Autodesk Fusion 360 part; units mm, degrees
(part 5 of 6)
  spline S27 degree 5 poles (67.7388, 69.1152) (67.7383, 69.1039) (67.7372, 69.0814) (67.7356, 69.0477) (67.7337, 69.0027) (67.7316, 68.9466) (67.7297, 68.8905) (67.728, 68.8344) (67.7266, 68.7785) (67.7254, 68.7226) (67.7245, 68.6668) (67.7239, 68.611) (67.7235, 68.5553) (67.7233, 68.4997) (67.7234, 68.4441) (67.7237, 68.3886) (67.7243, 68.3332) (67.7252, 68.2779) (67.7263, 68.2226) (67.7277, 68.1674) (67.7294, 68.1123) (67.7313, 68.0573) (67.7334, 68.0023) (67.7359, 67.9474) (67.7386, 67.8927) (67.7416, 67.838) (67.7448, 67.7833) (67.7484, 67.7288) (67.7522, 67.6744) (67.7562, 67.6201) (67.7606, 67.5658) (67.7652, 67.5117) (67.7702, 67.4576) (67.7754, 67.4037) (67.7809, 67.3498) (67.7867, 67.2961) (67.7928, 67.2424) (67.7992, 67.1889) (67.8059, 67.1355) (67.8129, 67.0822) (67.8202, 67.029) (67.8278, 66.9759) (67.8357, 66.923) (67.844, 66.8701) (67.8526, 66.8174) (67.8615, 66.7649) (67.8707, 66.7124) (67.8803, 66.6601) (67.8901, 66.6079) (67.9004, 66.5559) (67.9109, 66.504) (67.9219, 66.4523) (67.9333, 66.4007) (67.945, 66.3493) (67.9572, 66.2981) (67.9697, 66.247) (67.9825, 66.1961) (67.9957, 66.1454) (68.0093, 66.0948) (68.0233, 66.0444) (68.0378, 65.9942) (68.0528, 65.9443) (68.0685, 65.8947) (68.0848, 65.8454) (68.1017, 65.7964) (68.1189, 65.7475) (68.1365, 65.6989) (68.1543, 65.6503) (68.1726, 65.602) (68.1917, 65.5541) (68.212, 65.5069) (68.2297, 65.4698) (68.2439, 65.4424) (68.2539, 65.4245) (68.2589, 65.4155) knots -1 -1 -1 -1 -1 -1 -0.98571429 -0.97142857 -0.95714286 -0.94285714 -0.92857143 -0.91428571 -0.9 -0.88571429 -0.87142857 -0.85714286 -0.84285714 -0.82857143 -0.81428571 -0.8 -0.78571429 -0.77142857 -0.75714286 -0.74285714 -0.72857143 -0.71428571 -0.7 -0.68571429 -0.67142857 -0.65714286 -0.64285714 -0.62857143 -0.61428571 -0.6 -0.58571429 -0.57142857 -0.55714286 -0.54285714 -0.52857143 -0.51428571 -0.5 -0.48571429 -0.47142857 -0.45714286 -0.44285714 -0.42857143 -0.41428571 -0.4 -0.38571429 -0.37142857 -0.35714286 -0.34285714 -0.32857143 -0.31428571 -0.3 -0.28571429 -0.27142857 -0.25714286 -0.24285714 -0.22857143 -0.21428571 -0.2 -0.18571429 -0.17142857 -0.15714286 -0.14285714 -0.12857143 -0.11428571 -0.1 -0.08571429 -0.07142857 -0.05714286 -0.04285714 -0.02857143 -0.01428571 0 0 0 0 0 0
  line L29 (68.2589, 65.4155) -> (68.5051, 64.9824)
  arc A61 (68.3271, 64.3063) -> (68.5051, 64.9824) centre (68.0704, 64.7354) ccw
  arc A62 (68.3271, 64.3063) -> (67.3329, 63.6754) centre (79.882, 45) ccw
  arc A63 (66.6454, 63.8023) -> (67.3329, 63.6754) centre (67.0541, 64.0904) ccw
  line L30 (66.6454, 63.8023) -> (66.3584, 64.2094)
  spline S28 degree 5 poles (66.3584, 64.2094) (66.3524, 64.2178) (66.3404, 64.2344) (66.3217, 64.2589) (66.2957, 64.2907) (66.2616, 64.3293) (66.2264, 64.3669) (66.1905, 64.404) (66.1541, 64.4408) (66.1175, 64.4774) (66.0807, 64.5138) (66.0435, 64.55) (66.0058, 64.5857) (65.9676, 64.621) (65.9289, 64.6559) (65.8897, 64.6904) (65.85, 64.7245) (65.81, 64.7583) (65.7697, 64.7919) (65.7291, 64.8252) (65.6883, 64.8582) (65.6471, 64.891) (65.6056, 64.9235) (65.5638, 64.9558) (65.5216, 64.9877) (65.4792, 65.0194) (65.4365, 65.0508) (65.3935, 65.0819) (65.3502, 65.1129) (65.3067, 65.1435) (65.2629, 65.174) (65.2189, 65.2042) (65.1746, 65.2341) (65.1301, 65.2639) (65.0853, 65.2934) (65.0403, 65.3226) (64.995, 65.3516) (64.9495, 65.3804) (64.9038, 65.409) (64.8579, 65.4374) (64.8117, 65.4655) (64.7653, 65.4934) (64.7187, 65.5211) (64.6719, 65.5486) (64.6249, 65.5758) (64.5777, 65.6029) (64.5303, 65.6297) (64.4826, 65.6563) (64.4348, 65.6827) (64.3868, 65.7089) (64.3385, 65.7349) (64.2901, 65.7607) (64.2415, 65.7863) (64.1927, 65.8116) (64.1437, 65.8368) (64.0946, 65.8617) (64.0452, 65.8865) (63.9957, 65.911) (63.946, 65.9354) (63.8961, 65.9595) (63.8461, 65.9835) (63.7958, 66.0072) (63.7454, 66.0308) (63.6948, 66.0541) (63.6441, 66.0772) (63.5932, 66.1002) (63.5421, 66.1229) (63.4909, 66.1455) (63.4395, 66.1678) (63.3879, 66.19) (63.3362, 66.212) (63.2947, 66.2294) (63.2635, 66.2423) (63.2427, 66.2509) (63.2322, 66.2552) knots 0 0 0 0 0 0 0.01428571 0.02857143 0.04285714 0.05714286 0.07142857 0.08571429 0.1 0.11428571 0.12857143 0.14285714 0.15714286 0.17142857 0.18571429 0.2 0.21428571 0.22857143 0.24285714 0.25714286 0.27142857 0.28571429 0.3 0.31428571 0.32857143 0.34285714 0.35714286 0.37142857 0.38571429 0.4 0.41428571 0.42857143 0.44285714 0.45714286 0.47142857 0.48571429 0.5 0.51428571 0.52857143 0.54285714 0.55714286 0.57142857 0.58571429 0.6 0.61428571 0.62857143 0.64285714 0.65714286 0.67142857 0.68571429 0.7 0.71428571 0.72857143 0.74285714 0.75714286 0.77142857 0.78571429 0.8 0.81428571 0.82857143 0.84285714 0.85714286 0.87142857 0.88571429 0.9 0.91428571 0.92857143 0.94285714 0.95714286 0.97142857 0.98571429 1 1 1 1 1 1
  arc A64 (63.2322, 66.2552) -> (62.1231, 65.3377) centre (79.882, 45) ccw
  spline S29 degree 5 poles (62.1231, 65.3377) (62.1254, 65.3266) (62.1299, 65.3046) (62.1368, 65.2715) (62.1462, 65.2275) (62.158, 65.1725) (62.1701, 65.1177) (62.1825, 65.0631) (62.195, 65.0085) (62.2078, 64.9541) (62.2208, 64.8998) (62.234, 64.8456) (62.2475, 64.7915) (62.2612, 64.7376) (62.2751, 64.6838) (62.2892, 64.6302) (62.3036, 64.5766) (62.3182, 64.5233) (62.333, 64.47) (62.3481, 64.4169) (62.3634, 64.3639) (62.3789, 64.3111) (62.3947, 64.2584) (62.4107, 64.2059) (62.4269, 64.1535) (62.4434, 64.1013) (62.4601, 64.0492) (62.4771, 63.9972) (62.4943, 63.9455) (62.5118, 63.8938) (62.5295, 63.8424) (62.5475, 63.7911) (62.5657, 63.74) (62.5842, 63.689) (62.6029, 63.6382) (62.6219, 63.5876) (62.6411, 63.5372) (62.6606, 63.4869) (62.6804, 63.4368) (62.7004, 63.387) (62.7207, 63.3372) (62.7413, 63.2877) (62.7622, 63.2384) (62.7833, 63.1893) (62.8047, 63.1404) (62.8264, 63.0917) (62.8484, 63.0432) (62.8707, 62.9949) (62.8932, 62.9468) (62.9161, 62.899) (62.9392, 62.8513) (62.9627, 62.804) (62.9865, 62.7568) (63.0107, 62.71) (63.0352, 62.6634) (63.06, 62.6171) (63.0851, 62.5709) (63.1105, 62.5251) (63.1362, 62.4794) (63.1623, 62.4341) (63.1888, 62.3891) (63.2158, 62.3445) (63.2434, 62.3004) (63.2714, 62.2567) (63.2999, 62.2134) (63.3288, 62.1704) (63.3579, 62.1276) (63.3873, 62.085) (63.417, 62.0427) (63.4473, 62.0011) (63.4788, 61.9604) (63.5052, 61.9289) (63.5257, 61.9059) (63.5398, 61.891) (63.547, 61.8836) knots -1 -1 -1 -1 -1 -1 -0.98571429 -0.97142857 -0.95714286 -0.94285714 -0.92857143 -0.91428571 -0.9 -0.88571429 -0.87142857 -0.85714286 -0.84285714 -0.82857143 -0.81428571 -0.8 -0.78571429 -0.77142857 -0.75714286 -0.74285714 -0.72857143 -0.71428571 -0.7 -0.68571429 -0.67142857 -0.65714286 -0.64285714 -0.62857143 -0.61428571 -0.6 -0.58571429 -0.57142857 -0.55714286 -0.54285714 -0.52857143 -0.51428571 -0.5 -0.48571429 -0.47142857 -0.45714286 -0.44285714 -0.42857143 -0.41428571 -0.4 -0.38571429 -0.37142857 -0.35714286 -0.34285714 -0.32857143 -0.31428571 -0.3 -0.28571429 -0.27142857 -0.25714286 -0.24285714 -0.22857143 -0.21428571 -0.2 -0.18571429 -0.17142857 -0.15714286 -0.14285714 -0.12857143 -0.11428571 -0.1 -0.08571429 -0.07142857 -0.05714286 -0.04285714 -0.02857143 -0.01428571 0 0 0 0 0 0
  line L31 (63.547, 61.8836) -> (63.8931, 61.5253)
  arc A65 (63.8889, 60.8262) -> (63.8931, 61.5253) centre (63.5335, 61.1779) ccw
  arc A66 (63.8889, 60.8262) -> (63.0828, 59.9679) centre (79.882, 45) ccw
  arc A67 (62.3854, 59.9198) -> (63.0828, 59.9679) centre (62.7095, 60.3005) ccw
  line L32 (62.3854, 59.9198) -> (62.0061, 60.2427)
  spline S30 degree 5 poles (62.0061, 60.2427) (61.9982, 60.2493) (61.9824, 60.2625) (61.9582, 60.2816) (61.9251, 60.3059) (61.8825, 60.3347) (61.839, 60.3624) (61.795, 60.3894) (61.7507, 60.4161) (61.7061, 60.4424) (61.6614, 60.4685) (61.6164, 60.4943) (61.571, 60.5195) (61.5252, 60.5442) (61.479, 60.5684) (61.4325, 60.592) (61.3856, 60.6152) (61.3384, 60.638) (61.2911, 60.6605) (61.2435, 60.6826) (61.1957, 60.7045) (61.1476, 60.726) (61.0993, 60.7472) (61.0508, 60.768) (61.0021, 60.7885) (60.9531, 60.8086) (60.9039, 60.8284) (60.8545, 60.8479) (60.8049, 60.8671) (60.7551, 60.8859) (60.7051, 60.9045) (60.655, 60.9229) (60.6046, 60.9409) (60.5541, 60.9586) (60.5034, 60.976) (60.4525, 60.9931) (60.4015, 61.01) (60.3502, 61.0266) (60.2988, 61.0429) (60.2473, 61.0589) (60.1956, 61.0747) (60.1437, 61.0902) (60.0917, 61.1054) (60.0395, 61.1204) (59.9872, 61.1351) (59.9348, 61.1496) (59.8822, 61.1638) (59.8294, 61.1777) (59.7765, 61.1914) (59.7235, 61.2048) (59.6703, 61.218) (59.617, 61.2309) (59.5636, 61.2436) (59.51, 61.256) (59.4563, 61.2682) (59.4025, 61.2802) (59.3485, 61.2919) (59.2944, 61.3033) (59.2402, 61.3145) (59.1859, 61.3255) (59.1315, 61.3363) (59.0769, 61.3468) (59.0222, 61.357) (58.9675, 61.3671) (58.9125, 61.3769) (58.8575, 61.3864) (58.8024, 61.3957) (58.7472, 61.4048) (58.6918, 61.4137) (58.6364, 61.4224) (58.5808, 61.4308) (58.5363, 61.4373) (58.5028, 61.4421) (58.4805, 61.4453) (58.4694, 61.4468) knots 0 0 0 0 0 0 0.01428571 0.02857143 0.04285714 0.05714286 0.07142857 0.08571429 0.1 0.11428571 0.12857143 0.14285714 0.15714286 0.17142857 0.18571429 0.2 0.21428571 0.22857143 0.24285714 0.25714286 0.27142857 0.28571429 0.3 0.31428571 0.32857143 0.34285714 0.35714286 0.37142857 0.38571429 0.4 0.41428571 0.42857143 0.44285714 0.45714286 0.47142857 0.48571429 0.5 0.51428571 0.52857143 0.54285714 0.55714286 0.57142857 0.58571429 0.6 0.61428571 0.62857143 0.64285714 0.65714286 0.67142857 0.68571429 0.7 0.71428571 0.72857143 0.74285714 0.75714286 0.77142857 0.78571429 0.8 0.81428571 0.82857143 0.84285714 0.85714286 0.87142857 0.88571429 0.9 0.91428571 0.92857143 0.94285714 0.95714286 0.97142857 0.98571429 1 1 1 1 1 1
  arc A68 (58.4694, 61.4468) -> (57.6233, 60.2823) centre (79.882, 45) ccw
  spline S31 degree 5 poles (57.6233, 60.2823) (57.6282, 60.2722) (57.6381, 60.2519) (57.653, 60.2216) (57.673, 60.1813) (57.6982, 60.131) (57.7235, 60.0809) (57.7491, 60.0311) (57.7748, 59.9813) (57.8007, 59.9318) (57.8268, 59.8824) (57.8531, 59.8332) (57.8795, 59.7842) (57.9062, 59.7354) (57.933, 59.6868) (57.9601, 59.6383) (57.9873, 59.59) (58.0147, 59.5419) (58.0423, 59.4941) (58.0701, 59.4464) (58.0981, 59.3989) (58.1263, 59.3516) (58.1547, 59.3045) (58.1833, 59.2575) (58.212, 59.2108) (58.241, 59.1644) (58.2702, 59.1181) (58.2995, 59.072) (58.3291, 59.0261) (58.3588, 58.9805) (58.3888, 58.935) (58.4189, 58.8898) (58.4493, 58.8448) (58.4799, 58.8001) (58.5106, 58.7555) (58.5416, 58.7112) (58.5728, 58.6672) (58.6042, 58.6233) (58.6358, 58.5798) (58.6676, 58.5364) (58.6996, 58.4933) (58.7318, 58.4505) (58.7643, 58.4079) (58.797, 58.3656) (58.8299, 58.3235) (58.863, 58.2818) (58.8964, 58.2402) (58.93, 58.199) (58.9638, 58.158) (58.9978, 58.1174) (59.0321, 58.077) (59.0666, 58.0369) (59.1014, 57.9972) (59.1364, 57.9579) (59.1718, 57.9188) (59.2073, 57.8801) (59.2431, 57.8417) (59.2791, 57.8036) (59.3154, 57.7658) (59.3519, 57.7283) (59.3888, 57.6914) (59.426, 57.6549) (59.4637, 57.619) (59.5017, 57.5837) (59.5401, 57.5488) (59.5788, 57.5143) (59.6176, 57.4801) (59.6566, 57.4462) (59.6959, 57.4126) (59.7357, 57.3798) (59.7763, 57.3482) (59.8096, 57.3243) (59.8353, 57.3072) (59.8526, 57.2962) (59.8614, 57.2908) knots -1 -1 -1 -1 -1 -1 -0.98571429 -0.97142857 -0.95714286 -0.94285714 -0.92857143 -0.91428571 -0.9 -0.88571429 -0.87142857 -0.85714286 -0.84285714 -0.82857143 -0.81428571 -0.8 -0.78571429 -0.77142857 -0.75714286 -0.74285714 -0.72857143 -0.71428571 -0.7 -0.68571429 -0.67142857 -0.65714286 -0.64285714 -0.62857143 -0.61428571 -0.6 -0.58571429 -0.57142857 -0.55714286 -0.54285714 -0.52857143 -0.51428571 -0.5 -0.48571429 -0.47142857 -0.45714286 -0.44285714 -0.42857143 -0.41428571 -0.4 -0.38571429 -0.37142857 -0.35714286 -0.34285714 -0.32857143 -0.31428571 -0.3 -0.28571429 -0.27142857 -0.25714286 -0.24285714 -0.22857143 -0.21428571 -0.2 -0.18571429 -0.17142857 -0.15714286 -0.14285714 -0.12857143 -0.11428571 -0.1 -0.08571429 -0.07142857 -0.05714286 -0.04285714 -0.02857143 -0.01428571 0 0 0 0 0 0
  line L33 (59.8614, 57.2908) -> (60.2857, 57.0298)
  arc A69 (60.4555, 56.3517) -> (60.2857, 57.0298) centre (60.0238, 56.6039) ccw
  arc A70 (60.4555, 56.3517) -> (59.8882, 55.3198) centre (79.882, 45) ccw
  arc A71 (59.2247, 55.0998) -> (59.8882, 55.3198) centre (59.4439, 55.5491) ccw
  line L34 (59.2247, 55.0998) -> (58.777, 55.3182)
  spline S32 degree 5 poles (58.777, 55.3182) (58.7677, 55.3227) (58.7491, 55.3315) (58.721, 55.344) (58.6829, 55.3593) (58.6344, 55.3767) (58.5854, 55.3927) (58.5361, 55.4079) (58.4865, 55.4227) (58.4368, 55.4371) (58.387, 55.4513) (58.337, 55.465) (58.2867, 55.4782) (58.2362, 55.4907) (58.1855, 55.5026) (58.1345, 55.514) (58.0834, 55.5248) (58.032, 55.5351) (57.9805, 55.5451) (57.9289, 55.5547) (57.8772, 55.564) (57.8253, 55.5729) (57.7733, 55.5814) (57.7211, 55.5895) (57.6688, 55.5972) (57.6163, 55.6045) (57.5638, 55.6114) (57.5111, 55.618) (57.4582, 55.6243) (57.4053, 55.6302) (57.3523, 55.6358) (57.2992, 55.641) (57.2459, 55.646) (57.1926, 55.6506) (57.1391, 55.6548) (57.0856, 55.6588) (57.0319, 55.6624) (56.9782, 55.6657) (56.9244, 55.6687) (56.8705, 55.6715) (56.8165, 55.6739) (56.7624, 55.676) (56.7082, 55.6778) (56.654, 55.6793) (56.5996, 55.6806) (56.5452, 55.6815) (56.4907, 55.6822) (56.4362, 55.6826) (56.3815, 55.6827) (56.3268, 55.6825) (56.272, 55.682) (56.2172, 55.6813) (56.1623, 55.6803) (56.1073, 55.679) (56.0523, 55.6775) (55.9972, 55.6756) (55.942, 55.6735) (55.8868, 55.6712) (55.8315, 55.6686) (55.7761, 55.6657) (55.7207, 55.6626) (55.6653, 55.6592) (55.6098, 55.6555) (55.5542, 55.6516) (55.4986, 55.6474) (55.4429, 55.643) (55.3872, 55.6384) (55.3314, 55.6334) (55.2756, 55.6283) (55.2198, 55.6228) (55.1639, 55.6172) (55.1191, 55.6124) (55.0855, 55.6088) (55.0631, 55.6063) (55.0519, 55.605) knots 0 0 0 0 0 0 0.01428571 0.02857143 0.04285714 0.05714286 0.07142857 0.08571429 0.1 0.11428571 0.12857143 0.14285714 0.15714286 0.17142857 0.18571429 0.2 0.21428571 0.22857143 0.24285714 0.25714286 0.27142857 0.28571429 0.3 0.31428571 0.32857143 0.34285714 0.35714286 0.37142857 0.38571429 0.4 0.41428571 0.42857143 0.44285714 0.45714286 0.47142857 0.48571429 0.5 0.51428571 0.52857143 0.54285714 0.55714286 0.57142857 0.58571429 0.6 0.61428571 0.62857143 0.64285714 0.65714286 0.67142857 0.68571429 0.7 0.71428571 0.72857143 0.74285714 0.75714286 0.77142857 0.78571429 0.8 0.81428571 0.82857143 0.84285714 0.85714286 0.87142857 0.88571429 0.9 0.91428571 0.92857143 0.94285714 0.95714286 0.97142857 0.98571429 1 1 1 1 1 1
  arc A72 (55.0519, 55.605) -> (54.522, 54.2666) centre (79.882, 45) ccw
  spline S33 degree 5 poles (54.522, 54.2666) (54.5293, 54.2581) (54.544, 54.2409) (54.5659, 54.2152) (54.5953, 54.1811) (54.6322, 54.1387) (54.6692, 54.0966) (54.7063, 54.0546) (54.7436, 54.0128) (54.781, 53.9713) (54.8186, 53.93) (54.8563, 53.8888) (54.8941, 53.848) (54.9321, 53.8073) (54.9702, 53.7669) (55.0084, 53.7266) (55.0468, 53.6867) (55.0853, 53.6469) (55.1239, 53.6074) (55.1627, 53.5681) (55.2017, 53.5291) (55.2407, 53.4903) (55.2799, 53.4517) (55.3193, 53.4134) (55.3587, 53.3753) (55.3984, 53.3374) (55.4381, 53.2999) (55.478, 53.2625) (55.518, 53.2255) (55.5582, 53.1886) (55.5985, 53.1521) (55.639, 53.1158) (55.6796, 53.0798) (55.7203, 53.044) (55.7612, 53.0085) (55.8022, 52.9733) (55.8434, 52.9384) (55.8847, 52.9038) (55.9261, 52.8694) (55.9677, 52.8353) (56.0094, 52.8015) (56.0513, 52.7681) (56.0934, 52.7349) (56.1355, 52.702) (56.1779, 52.6695) (56.2203, 52.6373) (56.263, 52.6054) (56.3057, 52.5738) (56.3487, 52.5425) (56.3917, 52.5116) (56.435, 52.481) (56.4784, 52.4508) (56.522, 52.421) (56.5657, 52.3916) (56.6096, 52.3625) (56.6537, 52.3339) (56.6979, 52.3056) (56.7423, 52.2776) (56.7868, 52.25) (56.8315, 52.2228) (56.8764, 52.1962) (56.9215, 52.1701) (56.9669, 52.1447) (57.0126, 52.12) (57.0584, 52.0957) (57.1044, 52.0719) (57.1506, 52.0485) (57.1968, 52.0253) (57.2432, 52.0026) (57.2899, 51.9807) (57.337, 51.9602) (57.3753, 51.9453) (57.4044, 51.9351) (57.424, 51.9288) (57.4338, 51.9257) knots -1 -1 -1 -1 -1 -1 -0.98571429 -0.97142857 -0.95714286 -0.94285714 -0.92857143 -0.91428571 -0.9 -0.88571429 -0.87142857 -0.85714286 -0.84285714 -0.82857143 -0.81428571 -0.8 -0.78571429 -0.77142857 -0.75714286 -0.74285714 -0.72857143 -0.71428571 -0.7 -0.68571429 -0.67142857 -0.65714286 -0.64285714 -0.62857143 -0.61428571 -0.6 -0.58571429 -0.57142857 -0.55714286 -0.54285714 -0.52857143 -0.51428571 -0.5 -0.48571429 -0.47142857 -0.45714286 -0.44285714 -0.42857143 -0.41428571 -0.4 -0.38571429 -0.37142857 -0.35714286 -0.34285714 -0.32857143 -0.31428571 -0.3 -0.28571429 -0.27142857 -0.25714286 -0.24285714 -0.22857143 -0.21428571 -0.2 -0.18571429 -0.17142857 -0.15714286 -0.14285714 -0.12857143 -0.11428571 -0.1 -0.08571429 -0.07142857 -0.05714286 -0.04285714 -0.02857143 -0.01428571 0 0 0 0 0 0
  line L35 (57.4338, 51.9257) -> (57.9097, 51.7785)
  arc A73 (58.2428, 51.1639) -> (57.9097, 51.7785) centre (57.7619, 51.3008) ccw
  arc A74 (58.2428, 51.1639) -> (57.9499, 50.0233) centre (79.882, 45) ccw
  arc A75 (57.3619, 49.6452) -> (57.9499, 50.0233) centre (57.4626, 50.135) ccw
  line L36 (57.3619, 49.6452) -> (56.874, 49.7455)
  spline S34 degree 5 poles (56.874, 49.7455) (56.8639, 49.7475) (56.8437, 49.7514) (56.8133, 49.7565) (56.7726, 49.7619) (56.7214, 49.7666) (56.6699, 49.7699) (56.6183, 49.7724) (56.5667, 49.7744) (56.5149, 49.776) (56.4632, 49.7773) (56.4113, 49.7782) (56.3594, 49.7785) (56.3073, 49.7781) (56.2552, 49.777) (56.2031, 49.7753) (56.1508, 49.773) (56.0985, 49.7703) (56.0461, 49.7671) (55.9938, 49.7636) (55.9413, 49.7597) (55.8889, 49.7554) (55.8364, 49.7507) (55.7838, 49.7456) (55.7312, 49.7401) (55.6786, 49.7341) (55.626, 49.7277) (55.5733, 49.721) (55.5206, 49.7139) (55.4679, 49.7065) (55.4151, 49.6987) (55.3623, 49.6906) (55.3095, 49.6821) (55.2567, 49.6733) (55.2039, 49.6642) (55.151, 49.6547) (55.0982, 49.6448) (55.0453, 49.6347) (54.9924, 49.6242) (54.9395, 49.6135) (54.8866, 49.6024) (54.8337, 49.591) (54.7808, 49.5793) (54.7279, 49.5672) (54.6749, 49.5549) (54.622, 49.5423) (54.569, 49.5294) (54.5161, 49.5162) (54.4632, 49.5027) (54.4102, 49.4889) (54.3573, 49.4749) (54.3043, 49.4605) (54.2514, 49.4459) (54.1985, 49.431) (54.1455, 49.4158) (54.0926, 49.4003) (54.0397, 49.3846) (53.9868, 49.3686) (53.9339, 49.3523) (53.881, 49.3357) (53.8281, 49.3189) (53.7753, 49.3018) (53.7224, 49.2845) (53.6696, 49.2669) (53.6167, 49.249) (53.5639, 49.2309) (53.5111, 49.2125) (53.4583, 49.1939) (53.4055, 49.175) (53.3528, 49.1559) (53.3001, 49.1365) (53.2579, 49.1207) (53.2263, 49.1088) (53.2052, 49.1009) (53.1946, 49.0969) knots 0 0 0 0 0 0 0.01428571 0.02857143 0.04285714 0.05714286 0.07142857 0.08571429 0.1 0.11428571 0.12857143 0.14285714 0.15714286 0.17142857 0.18571429 0.2 0.21428571 0.22857143 0.24285714 0.25714286 0.27142857 0.28571429 0.3 0.31428571 0.32857143 0.34285714 0.35714286 0.37142857 0.38571429 0.4 0.41428571 0.42857143 0.44285714 0.45714286 0.47142857 0.48571429 0.5 0.51428571 0.52857143 0.54285714 0.55714286 0.57142857 0.58571429 0.6 0.61428571 0.62857143 0.64285714 0.65714286 0.67142857 0.68571429 0.7 0.71428571 0.72857143 0.74285714 0.75714286 0.77142857 0.78571429 0.8 0.81428571 0.82857143 0.84285714 0.85714286 0.87142857 0.88571429 0.9 0.91428571 0.92857143 0.94285714 0.95714286 0.97142857 0.98571429 1 1 1 1 1 1
  arc A76 (53.1946, 49.0969) -> (53.0142, 47.6687) centre (79.882, 45) ccw
  spline S35 degree 5 poles (53.0142, 47.6687) (53.0234, 47.6622) (53.0419, 47.6493) (53.0695, 47.6299) (53.1065, 47.6042) (53.1527, 47.5723) (53.1991, 47.5406) (53.2455, 47.5092) (53.292, 47.478) (53.3386, 47.4471) (53.3852, 47.4164) (53.4319, 47.3859) (53.4787, 47.3557) (53.5256, 47.3258) (53.5726, 47.2961) (53.6196, 47.2667) (53.6667, 47.2375) (53.7139, 47.2086) (53.7612, 47.1799) (53.8085, 47.1515) (53.8559, 47.1233) (53.9034, 47.0955) (53.951, 47.0679) (53.9986, 47.0405) (54.0463, 47.0135) (54.0941, 46.9867) (54.142, 46.9602) (54.1899, 46.9339) (54.2379, 46.908) (54.286, 46.8823) (54.3341, 46.8569) (54.3823, 46.8318) (54.4306, 46.807) (54.4789, 46.7825) (54.5273, 46.7583) (54.5758, 46.7344) (54.6244, 46.7108) (54.673, 46.6875) (54.7217, 46.6646) (54.7704, 46.6419) (54.8193, 46.6196) (54.8682, 46.5976) (54.9171, 46.5759) (54.9662, 46.5546) (55.0152, 46.5336) (55.0644, 46.5129) (55.1136, 46.4926) (55.1629, 46.4726) (55.2123, 46.453) (55.2617, 46.4338) (55.3112, 46.4149) (55.3607, 46.3965) (55.4103, 46.3784) (55.46, 46.3608) (55.5098, 46.3436) (55.5596, 46.3268) (55.6095, 46.3104) (55.6594, 46.2943) (55.7094, 46.2787) (55.7594, 46.2635) (55.8095, 46.2488) (55.8597, 46.2348) (55.91, 46.2215) (55.9604, 46.2089) (56.0108, 46.1968) (56.0613, 46.1852) (56.1118, 46.1739) (56.1624, 46.163) (56.213, 46.1525) (56.2636, 46.143) (56.3144, 46.1348) (56.3552, 46.1299) (56.3859, 46.1272) (56.4064, 46.126) (56.4167, 46.1255) knots -1 -1 -1 -1 -1 -1 -0.98571429 -0.97142857 -0.95714286 -0.94285714 -0.92857143 -0.91428571 -0.9 -0.88571429 -0.87142857 -0.85714286 -0.84285714 -0.82857143 -0.81428571 -0.8 -0.78571429 -0.77142857 -0.75714286 -0.74285714 -0.72857143 -0.71428571 -0.7 -0.68571429 -0.67142857 -0.65714286 -0.64285714 -0.62857143 -0.61428571 -0.6 -0.58571429 -0.57142857 -0.55714286 -0.54285714 -0.52857143 -0.51428571 -0.5 -0.48571429 -0.47142857 -0.45714286 -0.44285714 -0.42857143 -0.41428571 -0.4 -0.38571429 -0.37142857 -0.35714286 -0.34285714 -0.32857143 -0.31428571 -0.3 -0.28571429 -0.27142857 -0.25714286 -0.24285714 -0.22857143 -0.21428571 -0.2 -0.18571429 -0.17142857 -0.15714286 -0.14285714 -0.12857143 -0.11428571 -0.1 -0.08571429 -0.07142857 -0.05714286 -0.04285714 -0.02857143 -0.01428571 0 0 0 0 0 0
  line L37 (56.4167, 46.1255) -> (56.9142, 46.1012)
  arc A77 (57.3897, 45.5888) -> (56.9142, 46.1012) centre (56.8899, 45.6018) ccw
  arc A78 (57.3897, 45.5888) -> (57.3897, 44.4112) centre (79.882, 45) ccw
  arc A79 (56.9142, 43.8988) -> (57.3897, 44.4112) centre (56.8899, 44.3982) ccw
  line L38 (56.9142, 43.8988) -> (56.4167, 43.8745)
  spline S36 degree 5 poles (56.4167, 43.8745) (56.4064, 43.874) (56.3859, 43.8728) (56.3552, 43.8701) (56.3144, 43.8652) (56.2636, 43.857) (56.213, 43.8475) (56.1624, 43.837) (56.1118, 43.8261) (56.0613, 43.8148) (56.0108, 43.8032) (55.9604, 43.7911) (55.91, 43.7785) (55.8597, 43.7652) (55.8095, 43.7512) (55.7594, 43.7365) (55.7094, 43.7213) (55.6594, 43.7057) (55.6095, 43.6896) (55.5596, 43.6732) (55.5098, 43.6564) (55.46, 43.6392) (55.4103, 43.6216) (55.3607, 43.6035) (55.3112, 43.5851) (55.2617, 43.5662) (55.2123, 43.547) (55.1629, 43.5274) (55.1136, 43.5074) (55.0644, 43.4871) (55.0152, 43.4664) (54.9662, 43.4454) (54.9171, 43.4241) (54.8682, 43.4024) (54.8193, 43.3804) (54.7704, 43.3581) (54.7217, 43.3354) (54.673, 43.3125) (54.6244, 43.2892) (54.5758, 43.2656) (54.5273, 43.2417) (54.4789, 43.2175) (54.4306, 43.193) (54.3823, 43.1682) (54.3341, 43.1431) (54.286, 43.1177) (54.2379, 43.092) (54.1899, 43.0661) (54.142, 43.0398) (54.0941, 43.0133) (54.0463, 42.9865) (53.9986, 42.9595) (53.951, 42.9321) (53.9034, 42.9045) (53.8559, 42.8767) (53.8085, 42.8485) (53.7612, 42.8201) (53.7139, 42.7914) (53.6667, 42.7625) (53.6196, 42.7333) (53.5726, 42.7039) (53.5256, 42.6742) (53.4787, 42.6443) (53.4319, 42.6141) (53.3852, 42.5836) (53.3386, 42.5529) (53.292, 42.522) (53.2455, 42.4908) (53.1991, 42.4594) (53.1527, 42.4277) (53.1065, 42.3958) (53.0695, 42.3701) (53.0419, 42.3507) (53.0234, 42.3378) (53.0142, 42.3313) knots 0 0 0 0 0 0 0.01428571 0.02857143 0.04285714 0.05714286 0.07142857 0.08571429 0.1 0.11428571 0.12857143 0.14285714 0.15714286 0.17142857 0.18571429 0.2 0.21428571 0.22857143 0.24285714 0.25714286 0.27142857 0.28571429 0.3 0.31428571 0.32857143 0.34285714 0.35714286 0.37142857 0.38571429 0.4 0.41428571 0.42857143 0.44285714 0.45714286 0.47142857 0.48571429 0.5 0.51428571 0.52857143 0.54285714 0.55714286 0.57142857 0.58571429 0.6 0.61428571 0.62857143 0.64285714 0.65714286 0.67142857 0.68571429 0.7 0.71428571 0.72857143 0.74285714 0.75714286 0.77142857 0.78571429 0.8 0.81428571 0.82857143 0.84285714 0.85714286 0.87142857 0.88571429 0.9 0.91428571 0.92857143 0.94285714 0.95714286 0.97142857 0.98571429 1 1 1 1 1 1
  arc A80 (53.0142, 42.3313) -> (53.1946, 40.9031) centre (79.882, 45) ccw
  spline S37 degree 5 poles (53.1946, 40.9031) (53.2052, 40.8991) (53.2263, 40.8912) (53.2579, 40.8793) (53.3001, 40.8635) (53.3528, 40.8441) (53.4055, 40.825) (53.4583, 40.8061) (53.5111, 40.7875) (53.5639, 40.7691) (53.6167, 40.751) (53.6696, 40.7331) (53.7224, 40.7155) (53.7753, 40.6982) (53.8281, 40.6811) (53.881, 40.6643) (53.9339, 40.6477) (53.9868, 40.6314) (54.0397, 40.6154) (54.0926, 40.5997) (54.1455, 40.5842) (54.1985, 40.569) (54.2514, 40.5541) (54.3043, 40.5395) (54.3573, 40.5251) (54.4102, 40.5111) (54.4632, 40.4973) (54.5161, 40.4838) (54.569, 40.4706) (54.622, 40.4577) (54.6749, 40.4451) (54.7279, 40.4328) (54.7808, 40.4207) (54.8337, 40.409) (54.8866, 40.3976) (54.9395, 40.3865) (54.9924, 40.3758) (55.0453, 40.3653) (55.0982, 40.3552) (55.151, 40.3453) (55.2039, 40.3358) (55.2567, 40.3267) (55.3095, 40.3179) (55.3623, 40.3094) (55.4151, 40.3013) (55.4679, 40.2935) (55.5206, 40.2861) (55.5733, 40.279) (55.626, 40.2723) (55.6786, 40.2659) (55.7312, 40.2599) (55.7838, 40.2544) (55.8364, 40.2493) (55.8889, 40.2446) (55.9413, 40.2403) (55.9938, 40.2364) (56.0461, 40.2329) (56.0985, 40.2297) (56.1508, 40.227) (56.2031, 40.2247) (56.2552, 40.223) (56.3073, 40.2219) (56.3594, 40.2215) (56.4113, 40.2218) (56.4632, 40.2227) (56.5149, 40.224) (56.5667, 40.2256) (56.6183, 40.2276) (56.6699, 40.2301) (56.7214, 40.2334) (56.7726, 40.2381) (56.8133, 40.2435) (56.8437, 40.2486) (56.8639, 40.2525) (56.874, 40.2545) knots -1 -1 -1 -1 -1 -1 -0.98571429 -0.97142857 -0.95714286 -0.94285714 -0.92857143 -0.91428571 -0.9 -0.88571429 -0.87142857 -0.85714286 -0.84285714 -0.82857143 -0.81428571 -0.8 -0.78571429 -0.77142857 -0.75714286 -0.74285714 -0.72857143 -0.71428571 -0.7 -0.68571429 -0.67142857 -0.65714286 -0.64285714 -0.62857143 -0.61428571 -0.6 -0.58571429 -0.57142857 -0.55714286 -0.54285714 -0.52857143 -0.51428571 -0.5 -0.48571429 -0.47142857 -0.45714286 -0.44285714 -0.42857143 -0.41428571 -0.4 -0.38571429 -0.37142857 -0.35714286 -0.34285714 -0.32857143 -0.31428571 -0.3 -0.28571429 -0.27142857 -0.25714286 -0.24285714 -0.22857143 -0.21428571 -0.2 -0.18571429 -0.17142857 -0.15714286 -0.14285714 -0.12857143 -0.11428571 -0.1 -0.08571429 -0.07142857 -0.05714286 -0.04285714 -0.02857143 -0.01428571 0 0 0 0 0 0
  line L39 (56.874, 40.2545) -> (57.3619, 40.3548)
  arc A81 (57.9499, 39.9767) -> (57.3619, 40.3548) centre (57.4626, 39.865) ccw
  arc A82 (57.9499, 39.9767) -> (58.2428, 38.8361) centre (79.882, 45) ccw
  arc A83 (57.9097, 38.2215) -> (58.2428, 38.8361) centre (57.7619, 38.6992) ccw
  line L40 (57.9097, 38.2215) -> (57.4338, 38.0743)
  spline S38 degree 5 poles (57.4338, 38.0743) (57.424, 38.0712) (57.4044, 38.0649) (57.3753, 38.0547) (57.337, 38.0398) (57.2899, 38.0193) (57.2432, 37.9974) (57.1968, 37.9747) (57.1506, 37.9515) (57.1044, 37.9281) (57.0584, 37.9043) (57.0126, 37.88) (56.9669, 37.8553) (56.9215, 37.8299) (56.8764, 37.8038) (56.8315, 37.7772) (56.7868, 37.75) (56.7423, 37.7224) (56.6979, 37.6944) (56.6537, 37.6661) (56.6096, 37.6375) (56.5657, 37.6084) (56.522, 37.579) (56.4784, 37.5492) (56.435, 37.519) (56.3917, 37.4884) (56.3487, 37.4575) (56.3057, 37.4262) (56.263, 37.3946) (56.2203, 37.3627) (56.1779, 37.3305) (56.1355, 37.298) (56.0934, 37.2651) (56.0513, 37.2319) (56.0094, 37.1985) (55.9677, 37.1647) (55.9261, 37.1306) (55.8847, 37.0962) (55.8434, 37.0616) (55.8022, 37.0267) (55.7612, 36.9915) (55.7203, 36.956) (55.6796, 36.9202) (55.639, 36.8842) (55.5985, 36.8479) (55.5582, 36.8114) (55.518, 36.7745) (55.478, 36.7375) (55.4381, 36.7001) (55.3984, 36.6626) (55.3587, 36.6247) (55.3193, 36.5866) (55.2799, 36.5483) (55.2407, 36.5097) (55.2017, 36.4709) (55.1627, 36.4319) (55.1239, 36.3926) (55.0853, 36.3531) (55.0468, 36.3133) (55.0084, 36.2734) (54.9702, 36.2331) (54.9321, 36.1927) (54.8941, 36.152) (54.8563, 36.1112) (54.8186, 36.07) (54.781, 36.0287) (54.7436, 35.9872) (54.7063, 35.9454) (54.6692, 35.9034) (54.6322, 35.8613) (54.5953, 35.8189) (54.5659, 35.7848) (54.544, 35.7591) (54.5293, 35.7419) (54.522, 35.7334) knots 0 0 0 0 0 0 0.01428571 0.02857143 0.04285714 0.05714286 0.07142857 0.08571429 0.1 0.11428571 0.12857143 0.14285714 0.15714286 0.17142857 0.18571429 0.2 0.21428571 0.22857143 0.24285714 0.25714286 0.27142857 0.28571429 0.3 0.31428571 0.32857143 0.34285714 0.35714286 0.37142857 0.38571429 0.4 0.41428571 0.42857143 0.44285714 0.45714286 0.47142857 0.48571429 0.5 0.51428571 0.52857143 0.54285714 0.55714286 0.57142857 0.58571429 0.6 0.61428571 0.62857143 0.64285714 0.65714286 0.67142857 0.68571429 0.7 0.71428571 0.72857143 0.74285714 0.75714286 0.77142857 0.78571429 0.8 0.81428571 0.82857143 0.84285714 0.85714286 0.87142857 0.88571429 0.9 0.91428571 0.92857143 0.94285714 0.95714286 0.97142857 0.98571429 1 1 1 1 1 1
  arc A84 (54.522, 35.7334) -> (55.0519, 34.395) centre (79.882, 45) ccw
  spline S39 degree 5 poles (55.0519, 34.395) (55.0631, 34.3937) (55.0855, 34.3912) (55.1191, 34.3876) (55.1639, 34.3828) (55.2198, 34.3772) (55.2756, 34.3717) (55.3314, 34.3666) (55.3872, 34.3616) (55.4429, 34.357) (55.4986, 34.3526) (55.5542, 34.3484) (55.6098, 34.3445) (55.6653, 34.3408) (55.7207, 34.3374) (55.7761, 34.3343) (55.8315, 34.3314) (55.8868, 34.3288) (55.942, 34.3265) (55.9972, 34.3244) (56.0523, 34.3225) (56.1073, 34.321) (56.1623, 34.3197) (56.2172, 34.3187) (56.272, 34.318) (56.3268, 34.3175) (56.3815, 34.3173) (56.4362, 34.3174) (56.4907, 34.3178) (56.5452, 34.3185) (56.5996, 34.3194) (56.654, 34.3207) (56.7082, 34.3222) (56.7624, 34.324) (56.8165, 34.3261) (56.8705, 34.3285) (56.9244, 34.3313) (56.9782, 34.3343) (57.0319, 34.3376) (57.0856, 34.3412) (57.1391, 34.3452) (57.1926, 34.3494) (57.2459, 34.354) (57.2992, 34.359) (57.3523, 34.3642) (57.4053, 34.3698) (57.4582, 34.3757) (57.5111, 34.382) (57.5638, 34.3886) (57.6163, 34.3955) (57.6688, 34.4028) (57.7211, 34.4105) (57.7733, 34.4186) (57.8253, 34.4271) (57.8772, 34.436) (57.9289, 34.4453) (57.9805, 34.4549) (58.032, 34.4649) (58.0834, 34.4752) (58.1345, 34.486) (58.1855, 34.4974) (58.2362, 34.5093) (58.2867, 34.5218) (58.337, 34.535) (58.387, 34.5487) (58.4368, 34.5629) (58.4865, 34.5773) (58.5361, 34.5921) (58.5854, 34.6073) (58.6344, 34.6233) (58.6829, 34.6407) (58.721, 34.656) (58.7491, 34.6685) (58.7677, 34.6773) (58.777, 34.6818) knots -1 -1 -1 -1 -1 -1 -0.98571429 -0.97142857 -0.95714286 -0.94285714 -0.92857143 -0.91428571 -0.9 -0.88571429 -0.87142857 -0.85714286 -0.84285714 -0.82857143 -0.81428571 -0.8 -0.78571429 -0.77142857 -0.75714286 -0.74285714 -0.72857143 -0.71428571 -0.7 -0.68571429 -0.67142857 -0.65714286 -0.64285714 -0.62857143 -0.61428571 -0.6 -0.58571429 -0.57142857 -0.55714286 -0.54285714 -0.52857143 -0.51428571 -0.5 -0.48571429 -0.47142857 -0.45714286 -0.44285714 -0.42857143 -0.41428571 -0.4 -0.38571429 -0.37142857 -0.35714286 -0.34285714 -0.32857143 -0.31428571 -0.3 -0.28571429 -0.27142857 -0.25714286 -0.24285714 -0.22857143 -0.21428571 -0.2 -0.18571429 -0.17142857 -0.15714286 -0.14285714 -0.12857143 -0.11428571 -0.1 -0.08571429 -0.07142857 -0.05714286 -0.04285714 -0.02857143 -0.01428571 0 0 0 0 0 0
  line L41 (58.777, 34.6818) -> (59.2247, 34.9002)
  arc A85 (59.8882, 34.6802) -> (59.2247, 34.9002) centre (59.4439, 34.4509) ccw
  arc A86 (59.8882, 34.6802) -> (60.4555, 33.6483) centre (79.882, 45) ccw
  arc A87 (60.2857, 32.9702) -> (60.4555, 33.6483) centre (60.0238, 33.3961) ccw
  line L42 (60.2857, 32.9702) -> (59.8614, 32.7092)
  spline S40 degree 5 poles (59.8614, 32.7092) (59.8526, 32.7038) (59.8353, 32.6928) (59.8096, 32.6757) (59.7763, 32.6518) (59.7357, 32.6202) (59.6959, 32.5874) (59.6566, 32.5538) (59.6176, 32.5199) (59.5788, 32.4857) (59.5401, 32.4512) (59.5017, 32.4163) (59.4637, 32.381) (59.426, 32.3451) (59.3888, 32.3086) (59.3519, 32.2717) (59.3154, 32.2342) (59.2791, 32.1964) (59.2431, 32.1583) (59.2073, 32.1199) (59.1718, 32.0812) (59.1364, 32.0421) (59.1014, 32.0028) (59.0666, 31.9631) (59.0321, 31.923) (58.9978, 31.8826) (58.9638, 31.842) (58.93, 31.801) (58.8964, 31.7598) (58.863, 31.7182) (58.8299, 31.6765) (58.797, 31.6344) (58.7643, 31.5921) (58.7318, 31.5495) (58.6996, 31.5067) (58.6676, 31.4636) (58.6358, 31.4202) (58.6042, 31.3767) (58.5728, 31.3328) (58.5416, 31.2888) (58.5106, 31.2445) (58.4799, 31.1999) (58.4493, 31.1552) (58.4189, 31.1102) (58.3888, 31.065) (58.3588, 31.0195) (58.3291, 30.9739) (58.2995, 30.928) (58.2702, 30.8819) (58.241, 30.8356) (58.212, 30.7892) (58.1833, 30.7425) (58.1547, 30.6955) (58.1263, 30.6484) (58.0981, 30.6011) (58.0701, 30.5536) (58.0423, 30.5059) (58.0147, 30.4581) (57.9873, 30.41) (57.9601, 30.3617) (57.933, 30.3132) (57.9062, 30.2646) (57.8795, 30.2158) (57.8531, 30.1668) (57.8268, 30.1176) (57.8007, 30.0682) (57.7748, 30.0187) (57.7491, 29.9689) (57.7235, 29.9191) (57.6982, 29.869) (57.673, 29.8187) (57.653, 29.7784) (57.6381, 29.7481) (57.6282, 29.7278) (57.6233, 29.7177) knots 0 0 0 0 0 0 0.01428571 0.02857143 0.04285714 0.05714286 0.07142857 0.08571429 0.1 0.11428571 0.12857143 0.14285714 0.15714286 0.17142857 0.18571429 0.2 0.21428571 0.22857143 0.24285714 0.25714286 0.27142857 0.28571429 0.3 0.31428571 0.32857143 0.34285714 0.35714286 0.37142857 0.38571429 0.4 0.41428571 0.42857143 0.44285714 0.45714286 0.47142857 0.48571429 0.5 0.51428571 0.52857143 0.54285714 0.55714286 0.57142857 0.58571429 0.6 0.61428571 0.62857143 0.64285714 0.65714286 0.67142857 0.68571429 0.7 0.71428571 0.72857143 0.74285714 0.75714286 0.77142857 0.78571429 0.8 0.81428571 0.82857143 0.84285714 0.85714286 0.87142857 0.88571429 0.9 0.91428571 0.92857143 0.94285714 0.95714286 0.97142857 0.98571429 1 1 1 1 1 1
  arc A88 (57.6233, 29.7177) -> (58.4694, 28.5532) centre (79.882, 45) ccw
  spline S41 degree 5 poles (58.4694, 28.5532) (58.4805, 28.5547) (58.5028, 28.5579) (58.5363, 28.5627) (58.5808, 28.5692) (58.6364, 28.5776) (58.6918, 28.5863) (58.7472, 28.5952) (58.8024, 28.6043) (58.8575, 28.6136) (58.9125, 28.6231) (58.9675, 28.6329) (59.0222, 28.643) (59.0769, 28.6532) (59.1315, 28.6637) (59.1859, 28.6745) (59.2402, 28.6855) (59.2944, 28.6967) (59.3485, 28.7081) (59.4025, 28.7198) (59.4563, 28.7318) (59.51, 28.744) (59.5636, 28.7564) (59.617, 28.7691) (59.6703, 28.782) (59.7235, 28.7952) (59.7765, 28.8086) (59.8294, 28.8223) (59.8822, 28.8362) (59.9348, 28.8504) (59.9872, 28.8649) (60.0395, 28.8796) (60.0917, 28.8946) (60.1437, 28.9098) (60.1956, 28.9253) (60.2473, 28.9411) (60.2988, 28.9571) (60.3502, 28.9734) (60.4015, 28.99) (60.4525, 29.0069) (60.5034, 29.024) (60.5541, 29.0414) (60.6046, 29.0591) (60.655, 29.0771) (60.7051, 29.0955) (60.7551, 29.1141) (60.8049, 29.1329) (60.8545, 29.1521) (60.9039, 29.1716) (60.9531, 29.1914) (61.0021, 29.2115) (61.0508, 29.232) (61.0993, 29.2528) (61.1476, 29.274) (61.1957, 29.2955) (61.2435, 29.3174) (61.2911, 29.3395) (61.3384, 29.362) (61.3856, 29.3848) (61.4325, 29.408) (61.479, 29.4316) (61.5252, 29.4558) (61.571, 29.4805) (61.6164, 29.5057) (61.6614, 29.5315) (61.7061, 29.5576) (61.7507, 29.5839) (61.795, 29.6106) (61.839, 29.6376) (61.8825, 29.6653) (61.9251, 29.6941) (61.9582, 29.7184) (61.9824, 29.7375) (61.9982, 29.7507) (62.0061, 29.7573) knots -1 -1 -1 -1 -1 -1 -0.98571429 -0.97142857 -0.95714286 -0.94285714 -0.92857143 -0.91428571 -0.9 -0.88571429 -0.87142857 -0.85714286 -0.84285714 -0.82857143 -0.81428571 -0.8 -0.78571429 -0.77142857 -0.75714286 -0.74285714 -0.72857143 -0.71428571 -0.7 -0.68571429 -0.67142857 -0.65714286 -0.64285714 -0.62857143 -0.61428571 -0.6 -0.58571429 -0.57142857 -0.55714286 -0.54285714 -0.52857143 -0.51428571 -0.5 -0.48571429 -0.47142857 -0.45714286 -0.44285714 -0.42857143 -0.41428571 -0.4 -0.38571429 -0.37142857 -0.35714286 -0.34285714 -0.32857143 -0.31428571 -0.3 -0.28571429 -0.27142857 -0.25714286 -0.24285714 -0.22857143 -0.21428571 -0.2 -0.18571429 -0.17142857 -0.15714286 -0.14285714 -0.12857143 -0.11428571 -0.1 -0.08571429 -0.07142857 -0.05714286 -0.04285714 -0.02857143 -0.01428571 0 0 0 0 0 0
  line L43 (62.0061, 29.7573) -> (62.3854, 30.0802)
  arc A89 (63.0828, 30.0321) -> (62.3854, 30.0802) centre (62.7095, 29.6995) ccw
  arc A90 (63.0828, 30.0321) -> (63.8889, 29.1738) centre (79.882, 45) ccw
  arc A91 (63.8931, 28.4747) -> (63.8889, 29.1738) centre (63.5335, 28.8221) ccw
  line L44 (63.8931, 28.4747) -> (63.547, 28.1164)
  spline S42 degree 5 poles (63.547, 28.1164) (63.5398, 28.109) (63.5257, 28.0941) (63.5052, 28.0711) (63.4788, 28.0396) (63.4473, 27.9989) (63.417, 27.9573) (63.3873, 27.915) (63.3579, 27.8724) (63.3288, 27.8296) (63.2999, 27.7866) (63.2714, 27.7433) (63.2434, 27.6996) (63.2158, 27.6555) (63.1888, 27.6109) (63.1623, 27.5659) (63.1362, 27.5206) (63.1105, 27.4749) (63.0851, 27.4291) (63.06, 27.3829) (63.0352, 27.3366) (63.0107, 27.29) (62.9865, 27.2432) (62.9627, 27.196) (62.9392, 27.1487) (62.9161, 27.101) (62.8932, 27.0532) (62.8707, 27.0051) (62.8484, 26.9568) (62.8264, 26.9083) (62.8047, 26.8596) (62.7833, 26.8107) (62.7622, 26.7616) (62.7413, 26.7123) (62.7207, 26.6628) (62.7004, 26.613) (62.6804, 26.5632) (62.6606, 26.5131) (62.6411, 26.4628) (62.6219, 26.4124) (62.6029, 26.3618) (62.5842, 26.311) (62.5657, 26.26) (62.5475, 26.2089) (62.5295, 26.1576) (62.5118, 26.1062) (62.4943, 26.0545) (62.4771, 26.0028) (62.4601, 25.9508) (62.4434, 25.8987) (62.4269, 25.8465) (62.4107, 25.7941) (62.3947, 25.7416) (62.3789, 25.6889) (62.3634, 25.6361) (62.3481, 25.5831) (62.333, 25.53) (62.3182, 25.4767) (62.3036, 25.4234) (62.2892, 25.3698) (62.2751, 25.3162) (62.2612, 25.2624) (62.2475, 25.2085) (62.234, 25.1544) (62.2208, 25.1002) (62.2078, 25.0459) (62.195, 24.9915) (62.1825, 24.9369) (62.1701, 24.8823) (62.158, 24.8275) (62.1462, 24.7725) (62.1368, 24.7285) (62.1299, 24.6954) (62.1254, 24.6734) (62.1231, 24.6623) knots 0 0 0 0 0 0 0.01428571 0.02857143 0.04285714 0.05714286 0.07142857 0.08571429 0.1 0.11428571 0.12857143 0.14285714 0.15714286 0.17142857 0.18571429 0.2 0.21428571 0.22857143 0.24285714 0.25714286 0.27142857 0.28571429 0.3 0.31428571 0.32857143 0.34285714 0.35714286 0.37142857 0.38571429 0.4 0.41428571 0.42857143 0.44285714 0.45714286 0.47142857 0.48571429 0.5 0.51428571 0.52857143 0.54285714 0.55714286 0.57142857 0.58571429 0.6 0.61428571 0.62857143 0.64285714 0.65714286 0.67142857 0.68571429 0.7 0.71428571 0.72857143 0.74285714 0.75714286 0.77142857 0.78571429 0.8 0.81428571 0.82857143 0.84285714 0.85714286 0.87142857 0.88571429 0.9 0.91428571 0.92857143 0.94285714 0.95714286 0.97142857 0.98571429 1 1 1 1 1 1
  arc A92 (62.1231, 24.6623) -> (63.2322, 23.7448) centre (79.882, 45) ccw
  spline S43 degree 5 poles (63.2322, 23.7448) (63.2427, 23.7491) (63.2635, 23.7577) (63.2947, 23.7706) (63.3362, 23.788) (63.3879, 23.81) (63.4395, 23.8322) (63.4909, 23.8545) (63.5421, 23.8771) (63.5932, 23.8998) (63.6441, 23.9228) (63.6948, 23.9459) (63.7454, 23.9692) (63.7958, 23.9928) (63.8461, 24.0165) (63.8961, 24.0405) (63.946, 24.0646) (63.9957, 24.089) (64.0452, 24.1135) (64.0946, 24.1383) (64.1437, 24.1632) (64.1927, 24.1884) (64.2415, 24.2137) (64.2901, 24.2393) (64.3385, 24.2651) (64.3868, 24.2911) (64.4348, 24.3173) (64.4826, 24.3437) (64.5303, 24.3703) (64.5777, 24.3971) (64.6249, 24.4242) (64.6719, 24.4514) (64.7187, 24.4789) (64.7653, 24.5066) (64.8117, 24.5345) (64.8579, 24.5626) (64.9038, 24.591) (64.9495, 24.6196) (64.995, 24.6484) (65.0403, 24.6774) (65.0853, 24.7066) (65.1301, 24.7361) (65.1746, 24.7659) (65.2189, 24.7958) (65.2629, 24.826) (65.3067, 24.8565) (65.3502, 24.8871) (65.3935, 24.9181) (65.4365, 24.9492) (65.4792, 24.9806) (65.5216, 25.0123) (65.5638, 25.0442) (65.6056, 25.0765) (65.6471, 25.109) (65.6883, 25.1418) (65.7291, 25.1748) (65.7697, 25.2081) (65.81, 25.2417) (65.85, 25.2755) (65.8897, 25.3096) (65.9289, 25.3441) (65.9676, 25.379) (66.0058, 25.4143) (66.0435, 25.45) (66.0807, 25.4862) (66.1175, 25.5226) (66.1541, 25.5592) (66.1905, 25.596) (66.2264, 25.6331) (66.2616, 25.6707) (66.2957, 25.7093) (66.3217, 25.7411) (66.3404, 25.7656) (66.3524, 25.7822) (66.3584, 25.7906) knots -1 -1 -1 -1 -1 -1 -0.98571429 -0.97142857 -0.95714286 -0.94285714 -0.92857143 -0.91428571 -0.9 -0.88571429 -0.87142857 -0.85714286 -0.84285714 -0.82857143 -0.81428571 -0.8 -0.78571429 -0.77142857 -0.75714286 -0.74285714 -0.72857143 -0.71428571 -0.7 -0.68571429 -0.67142857 -0.65714286 -0.64285714 -0.62857143 -0.61428571 -0.6 -0.58571429 -0.57142857 -0.55714286 -0.54285714 -0.52857143 -0.51428571 -0.5 -0.48571429 -0.47142857 -0.45714286 -0.44285714 -0.42857143 -0.41428571 -0.4 -0.38571429 -0.37142857 -0.35714286 -0.34285714 -0.32857143 -0.31428571 -0.3 -0.28571429 -0.27142857 -0.25714286 -0.24285714 -0.22857143 -0.21428571 -0.2 -0.18571429 -0.17142857 -0.15714286 -0.14285714 -0.12857143 -0.11428571 -0.1 -0.08571429 -0.07142857 -0.05714286 -0.04285714 -0.02857143 -0.01428571 0 0 0 0 0 0
  line L45 (66.3584, 25.7906) -> (66.6454, 26.1977)
  arc A93 (67.3329, 26.3246) -> (66.6454, 26.1977) centre (67.0541, 25.9096) ccw
  arc A94 (67.3329, 26.3246) -> (68.3271, 25.6937) centre (79.882, 45) ccw
  arc A95 (68.5051, 25.0176) -> (68.3271, 25.6937) centre (68.0704, 25.2646) ccw
  line L46 (68.5051, 25.0176) -> (68.2589, 24.5845)
  spline S44 degree 5 poles (68.2589, 24.5845) (68.2539, 24.5755) (68.2439, 24.5576) (68.2297, 24.5302) (68.212, 24.4931) (68.1917, 24.4459) (68.1726, 24.398) (68.1543, 24.3497) (68.1365, 24.3011) (68.1189, 24.2525) (68.1017, 24.2036) (68.0848, 24.1546) (68.0685, 24.1053) (68.0528, 24.0557) (68.0378, 24.0058) (68.0233, 23.9556) (68.0093, 23.9052) (67.9957, 23.8546) (67.9825, 23.8039) (67.9697, 23.753) (67.9572, 23.7019) (67.945, 23.6507) (67.9333, 23.5993) (67.9219, 23.5477) (67.9109, 23.496) (67.9004, 23.4441) (67.8901, 23.3921) (67.8803, 23.3399) (67.8707, 23.2876) (67.8615, 23.2351) (67.8526, 23.1826) (67.844, 23.1299) (67.8357, 23.077) (67.8278, 23.0241) (67.8202, 22.971) (67.8129, 22.9178) (67.8059, 22.8645) (67.7992, 22.8111) (67.7928, 22.7576) (67.7867, 22.7039) (67.7809, 22.6502) (67.7754, 22.5963) (67.7702, 22.5424) (67.7652, 22.4883) (67.7606, 22.4342) (67.7562, 22.3799) (67.7522, 22.3256) (67.7484, 22.2712) (67.7448, 22.2167) (67.7416, 22.162) (67.7386, 22.1073) (67.7359, 22.0526) (67.7334, 21.9977) (67.7313, 21.9427) (67.7294, 21.8877) (67.7277, 21.8326) (67.7263, 21.7774) (67.7252, 21.7221) (67.7243, 21.6668) (67.7237, 21.6114) (67.7234, 21.5559) (67.7233, 21.5003) (67.7235, 21.4447) (67.7239, 21.389) (67.7245, 21.3332) (67.7254, 21.2774) (67.7266, 21.2215) (67.728, 21.1656) (67.7297, 21.1095) (67.7316, 21.0534) (67.7337, 20.9973) (67.7356, 20.9523) (67.7372, 20.9186) (67.7383, 20.8961) (67.7388, 20.8848) knots 0 0 0 0 0 0 0.01428571 0.02857143 0.04285714 0.05714286 0.07142857 0.08571429 0.1 0.11428571 0.12857143 0.14285714 0.15714286 0.17142857 0.18571429 0.2 0.21428571 0.22857143 0.24285714 0.25714286 0.27142857 0.28571429 0.3 0.31428571 0.32857143 0.34285714 0.35714286 0.37142857 0.38571429 0.4 0.41428571 0.42857143 0.44285714 0.45714286 0.47142857 0.48571429 0.5 0.51428571 0.52857143 0.54285714 0.55714286 0.57142857 0.58571429 0.6 0.61428571 0.62857143 0.64285714 0.65714286 0.67142857 0.68571429 0.7 0.71428571 0.72857143 0.74285714 0.75714286 0.77142857 0.78571429 0.8 0.81428571 0.82857143 0.84285714 0.85714286 0.87142857 0.88571429 0.9 0.91428571 0.92857143 0.94285714 0.95714286 0.97142857 0.98571429 1 1 1 1 1 1
  arc A96 (67.7388, 20.8848) -> (69.0413, 20.2719) centre (79.882, 45) ccw
  spline S45 degree 5 poles (69.0413, 20.2719) (69.0503, 20.2787) (69.0684, 20.2922) (69.0954, 20.3125) (69.1312, 20.3397) (69.1759, 20.3738) (69.2203, 20.4081) (69.2645, 20.4425) (69.3085, 20.4771) (69.3523, 20.5119) (69.3959, 20.5467) (69.4393, 20.5818) (69.4825, 20.617) (69.5255, 20.6523) (69.5682, 20.6878) (69.6108, 20.7234) (69.6531, 20.7592) (69.6952, 20.7952) (69.737, 20.8312) (69.7787, 20.8675) (69.8201, 20.9039) (69.8613, 20.9404) (69.9022, 20.9771) (69.943, 21.014) (69.9834, 21.051) (70.0237, 21.0882) (70.0637, 21.1255) (70.1034, 21.163) (70.143, 21.2006) (70.1822, 21.2384) (70.2212, 21.2763) (70.26, 21.3144) (70.2985, 21.3526) (70.3367, 21.3911) (70.3747, 21.4296) (70.4124, 21.4683) (70.4499, 21.5072) (70.487, 21.5463) (70.5239, 21.5855) (70.5606, 21.6249) (70.5969, 21.6644) (70.6329, 21.7041) (70.6687, 21.744) (70.7041, 21.784) (70.7392, 21.8242) (70.7741, 21.8646) (70.8086, 21.9051) (70.8428, 21.9458) (70.8767, 21.9867) (70.9103, 22.0277) (70.9435, 22.069) (70.9764, 22.1104) (71.0089, 22.152) (71.041, 22.1938) (71.0727, 22.2358) (71.1041, 22.278) (71.1351, 22.3204) (71.1658, 22.3629) (71.1962, 22.4056) (71.2261, 22.4485) (71.2555, 22.4916) (71.2843, 22.535) (71.3125, 22.5787) (71.3401, 22.6227) (71.3672, 22.667) (71.3938, 22.7114) (71.4202, 22.756) (71.4462, 22.8007) (71.4718, 22.8455) (71.4965, 22.8908) (71.5199, 22.9365) (71.5372, 22.9738) (71.5492, 23.0022) (71.5568, 23.0213) (71.5604, 23.0309) knots -1 -1 -1 -1 -1 -1 -0.98571429 -0.97142857 -0.95714286 -0.94285714 -0.92857143 -0.91428571 -0.9 -0.88571429 -0.87142857 -0.85714286 -0.84285714 -0.82857143 -0.81428571 -0.8 -0.78571429 -0.77142857 -0.75714286 -0.74285714 -0.72857143 -0.71428571 -0.7 -0.68571429 -0.67142857 -0.65714286 -0.64285714 -0.62857143 -0.61428571 -0.6 -0.58571429 -0.57142857 -0.55714286 -0.54285714 -0.52857143 -0.51428571 -0.5 -0.48571429 -0.47142857 -0.45714286 -0.44285714 -0.42857143 -0.41428571 -0.4 -0.38571429 -0.37142857 -0.35714286 -0.34285714 -0.32857143 -0.31428571 -0.3 -0.28571429 -0.27142857 -0.25714286 -0.24285714 -0.22857143 -0.21428571 -0.2 -0.18571429 -0.17142857 -0.15714286 -0.14285714 -0.12857143 -0.11428571 -0.1 -0.08571429 -0.07142857 -0.05714286 -0.04285714 -0.02857143 -0.01428571 0 0 0 0 0 0
  line L47 (71.5604, 23.0309) -> (71.7372, 23.4966)
  arc A97 (72.3716, 23.7905) -> (71.7372, 23.4966) centre (72.2047, 23.3192) ccw
  arc A98 (72.3716, 23.7905) -> (73.4915, 23.4266) centre (79.882, 45) ccw
  arc A99 (73.8319, 22.816) -> (73.4915, 23.4266) centre (73.3494, 22.9472) ccw
  line L48 (73.8319, 22.816) -> (73.7012, 22.3353)
  spline S46 degree 5 poles (73.7012, 22.3353) (73.6985, 22.3254) (73.6934, 22.3055) (73.6864, 22.2755) (73.6785, 22.2352) (73.6705, 22.1844) (73.664, 22.1332) (73.6583, 22.0819) (73.6531, 22.0304) (73.6482, 21.9789) (73.6436, 21.9273) (73.6395, 21.8756) (73.636, 21.8238) (73.6331, 21.7719) (73.6309, 21.7198) (73.6294, 21.6676) (73.6283, 21.6153) (73.6278, 21.5629) (73.6276, 21.5105) (73.6278, 21.458) (73.6284, 21.4054) (73.6294, 21.3528) (73.6308, 21.3001) (73.6326, 21.2473) (73.6349, 21.1945) (73.6375, 21.1416) (73.6406, 21.0887) (73.644, 21.0357) (73.6477, 20.9826) (73.6518, 20.9295) (73.6563, 20.8764) (73.6611, 20.8232) (73.6662, 20.77) (73.6717, 20.7167) (73.6775, 20.6634) (73.6837, 20.6101) (73.6901, 20.5567) (73.697, 20.5033) (73.7041, 20.4499) (73.7115, 20.3964) (73.7193, 20.3429) (73.7273, 20.2894) (73.7357, 20.2358) (73.7443, 20.1823) (73.7533, 20.1287) (73.7626, 20.075) (73.7721, 20.0214) (73.782, 19.9677) (73.7921, 19.914) (73.8026, 19.8603) (73.8133, 19.8066) (73.8243, 19.7529) (73.8355, 19.6991) (73.8471, 19.6454) (73.8589, 19.5916) (73.8711, 19.5378) (73.8834, 19.484) (73.8961, 19.4302) (73.909, 19.3764) (73.9222, 19.3225) (73.9357, 19.2687) (73.9494, 19.2149) (73.9634, 19.161) (73.9776, 19.1072) (73.9922, 19.0533) (74.0069, 18.9995) (74.022, 18.9456) (74.0372, 18.8918) (74.0528, 18.8379) (74.0686, 18.7841) (74.0846, 18.7302) (74.0977, 18.6871) (74.1076, 18.6548) (74.1142, 18.6333) (74.1175, 18.6225) knots 0 0 0 0 0 0 0.01428571 0.02857143 0.04285714 0.05714286 0.07142857 0.08571429 0.1 0.11428571 0.12857143 0.14285714 0.15714286 0.17142857 0.18571429 0.2 0.21428571 0.22857143 0.24285714 0.25714286 0.27142857 0.28571429 0.3 0.31428571 0.32857143 0.34285714 0.35714286 0.37142857 0.38571429 0.4 0.41428571 0.42857143 0.44285714 0.45714286 0.47142857 0.48571429 0.5 0.51428571 0.52857143 0.54285714 0.55714286 0.57142857 0.58571429 0.6 0.61428571 0.62857143 0.64285714 0.65714286 0.67142857 0.68571429 0.7 0.71428571 0.72857143 0.74285714 0.75714286 0.77142857 0.78571429 0.8 0.81428571 0.82857143 0.84285714 0.85714286 0.87142857 0.88571429 0.9 0.91428571 0.92857143 0.94285714 0.95714286 0.97142857 0.98571429 1 1 1 1 1 1
  arc A100 (74.1175, 18.6225) -> (75.5315, 18.3528) centre (79.882, 45) ccw